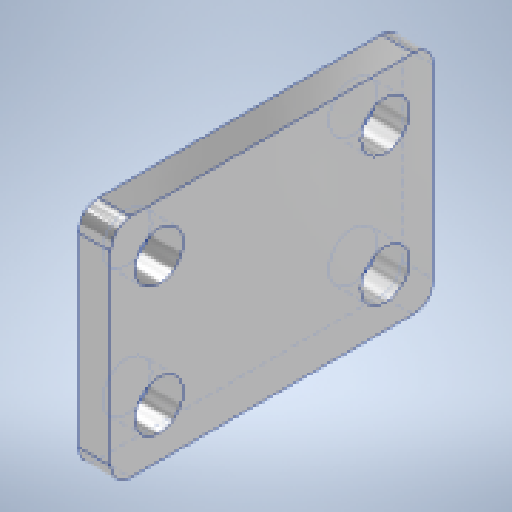
# Autodesk Inventor part: belt_holder_2
Saved by Autodesk Inventor 2025 (Build 290162000, 162)
## iProperties
Created: 2025-02-25
Part Number: belt_holder_2
Material: アルミニウム 6061
Document SubType Name: Modeling
Designer: Zhopa
Density: 2.7 g/cm^3
Appearance: アルミニウム - フラット
Mass: 1.35208 g
Surface Area: 7.07875 cm^2
Volume: 0.500769 cm^3
Author: Zhopa
Autodesk Inventor part; units mm, degrees
ref_plane "YZ Plane" through (0, 0, 0) normal (1, 0, 0) x (0, 1, 0)
ref_plane "XZ Plane" through (0, 0, 0) normal (0, 1, 0) x (-1, 0, 0)
ref_plane "XY Plane" through (0, 0, 0) normal (0, 0, 1) x (1, 0, 0)
sketch "Sketch1" plane through (0, 0, 0) normal (1, 0, 0) x (0, 1, 0)
  line L0 (0, 0) -> (14, 0)
  line L1 (14, 0) -> (14, -20)
  line L2 (14, -20) -> (0, -20)
  line L3 (0, -20) -> (0, 0)
  line L4 (14, -10) -> (0, -10)
  point P0 (11, -3)
  point P1 (3, -3)
  point P2 (11, -17)
  point P3 (3, -17)
  dimension "d0" = 14
  dimension "d1" = 20
  dimension "d2" = 8
  dimension "d3" = 3
  dimension "d4" = 3
  dimension "d5" = 3
  constraints: 10 end point, 2 midpoint, 2 parallel, 2 symmetric about line, 1 horizontal, 1 perpendicular
  measures "d0" distance of L1.end L2.end
  measures "d1" distance of L0.end L1.end
  measures "d2" distance of point (3, -3) point (11, -3)
  measures "d3" distance from line of L0 point (11, -3)
  measures "d4" distance from line of L0 point (3, -3)
  measures "d5" distance from line of L1 point (11, -3)
extrude "Extrusion1" add sketch "Sketch1" along normal blind 2
hole "Hole1" at (0, 11, -3) at (0, 3, -3) at (0, 11, -17) at (0, 3, -17) direction (1, 0, 0) diameter 3 depth 80.45
fillet "Fillet1" radius 1.25 4 edges at (1, 14, 0) (1, 14, -20) (1, 0, -20) (1, 0, 0)
body "Solid1"
